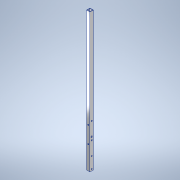
# Autodesk Inventor part: ハンド9x9_4_CPY
Saved by Autodesk Inventor 2020.3 (Build 243373000, 373)
## iProperties
Created: 2020-05-31
Part Number: ハンド9x9_4_CPY
Material: アルミニウム 6061
Document SubType Name: Modeling
Designer: totot
Mass: 32.004 g
Surface Area: 200.053 cm^2
Volume: 11.8533 cm^3
Density: 2.7 g/cm^3
Appearance: アルミニウム - フラット
Author: totot
Autodesk Inventor part; units mm, degrees
ref_plane "YZ Plane" through (0, 0, 0) normal (1, 0, 0) x (0, 1, 0)
ref_plane "XZ Plane" through (0, 0, 0) normal (0, 1, 0) x (-1, 0, 0)
ref_plane "XY Plane" through (0, 0, 0) normal (0, 0, 1) x (1, 0, 0)
sketch "スケッチ1" plane through (0, 0, 0) normal (0, 1, 0) x (-1, 0, 0)
  line L0 (0, 0) -> (-9, 0)
  line L1 (-9, 0) -> (-9, -9)
  line L2 (-9, -9) -> (0, -9)
  line L3 (0, -9) -> (0, 0)
  line L4 (-1.2, -1.2) -> (-7.8, -1.2)
  line L5 (-7.8, -1.2) -> (-7.8, -7.8)
  line L6 (-7.8, -7.8) -> (-1.2, -7.8)
  line L7 (-1.2, -7.8) -> (-1.2, -1.2)
  dimension "d0" = 9
  dimension "d1" = 9
  dimension "d2" = 1.2
  dimension "d3" = 1.2
  dimension "d4" = 1.2
  dimension "d5" = 1.2
  constraints: 16 end point, 4 parallel, 2 horizontal, 2 perpendicular
  measures "d0" distance of L0.start L0.end
  measures "d1" distance of L2.end L0.start
  measures "d2" distance between parallel lines of L0 L4
  measures "d3" distance between parallel lines of L7 L3
  measures "d4" distance between parallel lines of L6 L2
  measures "d5" distance between parallel lines of L1 L5
extrude "押し出し1" add sketch "スケッチ1" along normal blind 63
sketch "スケッチ2" plane through (9, 0, 0) normal (1, 0, 0) x (0, 0, -1)
  line L0 (0, 63) -> (9, 63) projected
  line L1 (9, 0) -> (9, 63) projected
  line L2 (0, 0) -> (9, 0) projected
  point P0 (4.5, 58.5)
  point P1 (4.5, 13.5)
  dimension "d8" = 4.5
  dimension "d9" = 4.5
  dimension "d10" = 4.5
  dimension "d11" = 13.5
  measures "d8" distance from line of point (4.5, 58.5) L0
  measures "d9" distance from line of point (4.5, 58.5) L1
  measures "d10" distance from line of L1 point (4.5, 13.5)
  measures "d11" distance from line of L2 point (4.5, 13.5)
hole "穴1" at (9, 58.5, -4.5) at (9, 13.5, -4.5) direction (-1, 0, 0) diameter 3.3 end through all
sketch "スケッチ3" plane through (0, 0, 0) normal (0, 0, 1) x (1, 0, 0)
  line L0 (0, 0) -> (0, 63) projected
  line L1 (0, 0) -> (9, 0) projected
  line L2 (0, 63) -> (9, 63) projected
  point P0 (4.5, 49.5)
  point P1 (4.5, 4.5)
  dimension "d19" = 4.5
  dimension "d20" = 4.5
  dimension "d21" = 13.5
  dimension "d22" = 4.5
  measures "d19" distance from line of L0 point (4.5, 4.5)
  measures "d20" distance from line of point (4.5, 4.5) L1
  measures "d21" distance from line of point (4.5, 49.5) L2
  measures "d22" distance from line of L0 point (4.5, 49.5)
hole "穴2" at (4.5, 49.5, 0) at (4.5, 4.5, 0) direction (0, 0, -1) diameter 3.3 end through all
sketch "スケッチ4" plane through (9, 0, 0) normal (1, 0, 0) x (0, 0, -1)
  line L0 (0, 0) -> (9, 0) projected
  line L1 (9, 0) -> (9, 63) projected
  point P0 (4.5, 22)
  dimension "d30" = 22
  dimension "d31" = 4.5
  measures "d30" distance from line of point (4.5, 22) L0
  measures "d31" distance from line of point (4.5, 22) L1
hole "穴3" at (9, 22, -4.5) direction (-1, 0, 0) diameter 4 end through all
sketch "スケッチ5" plane through (0, 63, 0) normal (0, 1, 0) x (1, 0, 0)
  line L0 (0, 9) -> (0, 0) projected
  line L1 (9, 0) -> (9, 9) projected
  line L2 (0, 0) -> (9, 0)
  line L3 (9, 0) -> (9, 9)
  line L4 (9, 9) -> (0, 9)
  line L5 (0, 9) -> (0, 0)
  line L6 (1.2, 1.2) -> (1.2, 7.8) projected
  line L7 (1.2, 7.8) -> (7.8, 7.8) projected
  line L8 (1.2, 1.2) -> (7.8, 1.2)
  line L9 (7.8, 1.2) -> (7.8, 7.8)
  line L10 (7.8, 7.8) -> (1.2, 7.8)
  line L11 (1.2, 7.8) -> (1.2, 1.2)
  constraints: 16 end point, 4 parallel, 2 horizontal, 2 perpendicular
extrude "押し出し2" add sketch "スケッチ5" along normal blind 200
sketch "スケッチ6" plane through (0, 0, 0) normal (0, -1, 0) x (1, 0, 0)
  line L0 (0, -9) -> (0, 0) projected
  line L1 (9, 0) -> (9, -9) projected
  line L2 (0, 0) -> (9, 0)
  line L3 (9, 0) -> (9, -9)
  line L4 (9, -9) -> (0, -9)
  line L5 (0, -9) -> (0, 0)
  line L6 (1.2, -1.2) -> (1.2, -7.8) projected
  line L7 (7.8, -7.8) -> (7.8, -1.2) projected
  line L8 (1.2, -1.2) -> (7.8, -1.2)
  line L9 (7.8, -1.2) -> (7.8, -7.8)
  line L10 (7.8, -7.8) -> (1.2, -7.8)
  line L11 (1.2, -7.8) -> (1.2, -1.2)
  constraints: 16 end point, 4 parallel, 2 horizontal, 2 perpendicular
extrude "押し出し3" add sketch "スケッチ6" along normal blind 57.5
sketch "スケッチ7" plane through (0, 263, -9) normal (-1, 0, 0) x (0, 0, 1)
  line L0 (0, -320.5) -> (0, 0) projected
  line L1 (9, -320.5) -> (0, -320.5) projected
  point P0 (9, -263)
  point P1 (4.5, -316)
  point P2 (4.5, -286)
  dimension "d43" = 4.5
  dimension "d44" = 4.5
  dimension "d45" = 4.5
  dimension "d46" = 30
  measures "d43" distance from line of L0 point (4.5, -286)
  measures "d44" distance from line of L0 point (4.5, -316)
  measures "d45" distance from line of L1 point (4.5, -316)
  measures "d46" distance of point (4.5, -316) point (4.5, -286)
hole "穴4" at (0, -53, -4.5) at (0, -23, -4.5) direction (1, 0, 0) diameter 3 end through all
sketch "スケッチ8" plane through (0, 263, 0) normal (0, 1, 0) x (1, 0, 0)
  line L0 (0, 0) -> (9, 0)
  line L1 (9, 0) -> (9, 9)
  line L2 (9, 9) -> (0, 9)
  line L3 (0, 9) -> (0, 0)
  line L4 (7.8, 7.8) -> (1.2, 7.8)
  line L5 (1.2, 7.8) -> (1.2, 1.2)
  line L6 (1.2, 1.2) -> (7.8, 1.2)
  line L7 (7.8, 1.2) -> (7.8, 7.8)
  constraints: 16 end point, 4 parallel, 2 horizontal, 2 perpendicular
extrude "押し出し4" add sketch "スケッチ8" along normal blind 50
equation "\"d4\" = d3"
equation "\"d5\" = d4"
equation "\"d9\" = d8"
equation "\"d10\" = d9"
equation "\"d20\" = d19"
equation "\"d22\" = d19"
